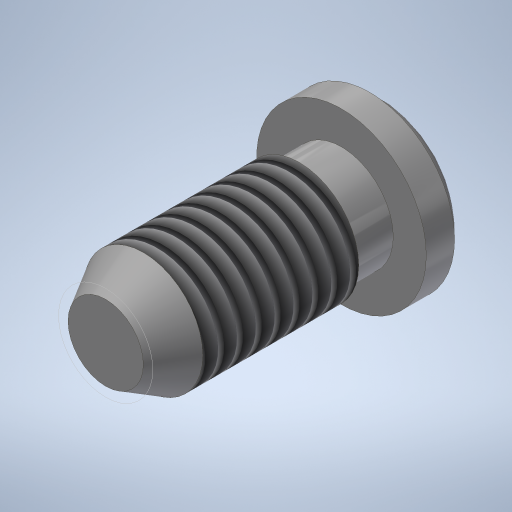
# Autodesk Inventor part: EuroScrew D9 L16 H
Saved by Autodesk Inventor 2024 (Build 280153000, 153)
## iProperties
Created: 2014-10-14
Part Number: EuroScrew D9 L16 H
Material: Generic
Document SubType Name: Modeling
Designer: G. Kazokaitis
Density: 1 g/cm^3
Appearance: Default
Author: G. Kazokaitis
Autodesk Inventor part; units mm, degrees
ref_plane "YZ Plane" through (0, 0, 0) normal (1, 0, 0) x (0, 1, 0)
ref_plane "XZ Plane" through (0, 0, 0) normal (0, 1, 0) x (-1, 0, 0)
ref_plane "XY Plane" through (0, 0, 0) normal (0, 0, 1) x (1, 0, 0)
sketch "Sketch1" plane through (0, 0, 0) normal (0, 0, 1) x (1, 0, 0)
  line L0 (3.15, -10.5612) -> (3.15, -2.2892)
  line L1 (1.997, -12.5582) -> (3.15, -10.5612)
  line L2 (0, -12.5582) -> (1.997, -12.5582)
  line L3 (0, -20.7284) -> (0, -13.6389) construction
  line L4 (0, -12.5582) -> (0, 3.4418)
  line L5 (2.6537, 0) -> (-1.8059, 0)
  line L6 (2.75, -2.0582) -> (2.75, -0.0582)
  line L7 (2.75, -0.0582) -> (4.5, -0.0582)
  line L8 (7.0831, -0.0582) -> (2.8831, -0.0582)
  arc A0 (4.5, 1.4418) -> (0, 3.4418) centre (0, -2.6207) ccw
  line L9 (4.5, -0.0582) -> (4.5, 1.4418)
  line L10 (3.15, -2.2892) -> (2.75, -2.0582)
  point P0 (0, 0)
  point P1 (0, -3.5)
  point P2 (0, -3.5)
  point P3 (0, 0.0007)
  point P4 (0.4239, 0)
  dimension "d0" = 6.3
  dimension "d1" = 5.5
  dimension "d2" = 2
  dimension "d4" = 16
  dimension "d5" = 9
  dimension "d6" = 1.5
  dimension "d7" = 30
  dimension "d8" = 1.153
  dimension "d9" = 3.4418
  constraints: 22 end point, 4 parallel, 4 point on line, 2 collinear, 2 perpendicular, 2 point on circle, 1 centre point, 1 horizontal, 1 midpoint, 1 vertical
  measures "d0" diameter of L0 L4
  measures "d1" diameter of L6 L4
  measures "d2" distance of L10.end L6.end
  measures "d4" distance of L2.start L4.end
  measures "d5" diameter of L9 L4
  measures "d6" distance of L7.end L9.end
  measures "d7" angle of L4 L1
  measures "d8" horizontal distance of L1.start L1.end
  measures "d9" distance from line of L4.end L5
revolve "Revolution1" add sketch "Sketch1" angle 360 about axis through (0, -12.5582, 0) along (0, 1, 0)
sketch "Sketch2" plane through (0, 0, 0) normal (0, 0, 1) x (1, 0, 0)
  line L0 (-0.6, 3.4418) -> (0.6, 3.4418)
  line L1 (0.6, 3.4418) -> (0.6, 1.4418)
  line L2 (0.6, 1.4418) -> (-0.6, 1.4418)
  line L3 (-0.6, 1.4418) -> (-0.6, 3.4418)
  arc A0 (4.5, 1.4418) -> (-4.5, 1.4418) centre (0, -2.6207) ccw projected
  point P0 (0, 0)
  point P1 (0, 3.4418)
  dimension "d11" = 1.2
  dimension "d12" = 2
  constraints: 8 end point, 2 parallel, 1 horizontal, 1 midpoint, 1 perpendicular, 1 point on circle, 1 tangent, 1 other
  measures "d11" distance of L1.end L2.end
  measures "d12" distance of L0.end L1.end
extrude "Extrusion1" cut sketch "Sketch2" along normal through all both and the other way through all
sketch "Sketch3" plane through (0, 0, 0) normal (0, 0, 1) x (1, 0, 0)
  line L0 (-2.2353, 3.7038) -> (2.2353, 3.7038)
  line L1 (2.2353, 3.7038) -> (1.666, 1.0827)
  line L2 (1.666, 1.0827) -> (-1.666, 1.0827)
  line L3 (-1.666, 1.0827) -> (-2.2353, 3.7038)
  point P0 (0, 0)
  point P1 (0, 3.7038)
  point P2 (0, 1.0827)
  constraints: 8 end point, 2 midpoint, 2 vertical alignment, 1 horizontal, 1 parallel
extrude "Extrusion2" cut sketch "Sketch3" along normal mid plane 1.2
thread "Thread1" size "M7x1" class "6g" standard "ISO Metric profile" full length
sketch "Sketch4" plane through (0, 1.4418, 0) normal (0, 1, 0) x (1, 0, 0)
  arc A0 (-0.6, -4.4598) -> (0.6, -4.4598) centre (0, 0) ccw projected
  circle A1 centre (0, 0) radius 2.5
  point P0 (-0.6, -3.4482)
  point P1 (0.6, -3.4482)
  dimension "d19" = 5
  constraints: 1 centre point, 1 coincident, 1 other
  measures "d19" diameter of A1
extrude "Extrusion3" add sketch "Sketch4" against normal up to surface (14 mm away) separate body
equation "\"d0\" = Thread_diameter"
equation "\"d4\" = Length"
equation "\"d5\" = Head_Diameter"
equation "\"Head_Diameter\" = 9"
equation "\"Thread_diameter\" = 6.3"
equation "\"Length\" = 16"
